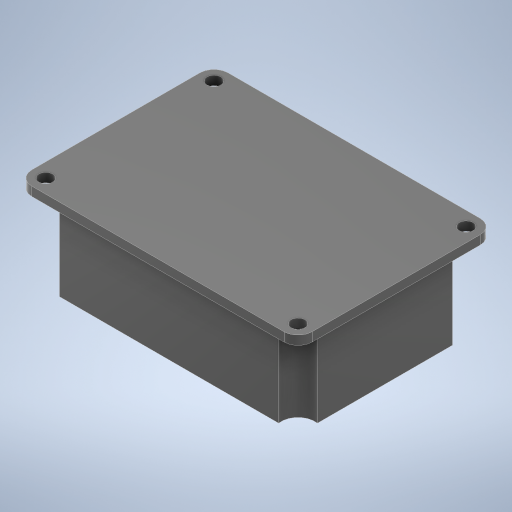
# Autodesk Inventor part: SUSTAINA-USB-AUDIO-BOARD
Saved by Autodesk Inventor 2024.2 (Build 282272000, 272)
## iProperties
Created: 2024-02-11
Part Number: SUSTAINA-USB-AUDIO-BOARD
Material: CFRP
Document SubType Name: Modeling
Designer: Masato Kubotera
Density: 1.43 g/cm^3
Appearance: Smooth - Black
Mass: 33.6504 g
Surface Area: 60.0346 cm^2
Volume: 23.5317 cm^3
Author: Masato Kubotera
Autodesk Inventor part; units mm, degrees
ref_plane "YZ Plane" through (0, 0, 0) normal (1, 0, 0) x (0, 1, 0)
ref_plane "XZ Plane" through (0, 0, 0) normal (0, 1, 0) x (-1, 0, 0)
ref_plane "XY Plane" through (0, 0, 0) normal (0, 0, 1) x (1, 0, 0)
sketch "Sketch1" plane through (0, 0, 0) normal (0, 0, 1) x (1, 0, 0)
  line L0 (17.5, 25) -> (-17.5, 25)
  line L1 (-17.5, 25) -> (-17.5, -25)
  line L2 (-17.5, -25) -> (17.5, -25)
  line L3 (17.5, -25) -> (17.5, 25)
  line L4 (17.5, 25) -> (-17.5, -25) construction
  line L5 (-17.5, 25) -> (17.5, -25) construction
  line L6 (-14, -18) -> (14, -18) construction
  line L7 (14, -18) -> (14, 18) construction
  line L8 (14, 18) -> (-14, 18) construction
  line L9 (-14, 18) -> (-14, -18) construction
  line L10 (-14, -18) -> (14, 18) construction
  line L11 (14, -18) -> (-14, 18) construction
  circle A0 centre (14, 18) radius 2.4 construction
  arc A1 (13.2801, 15.7105) -> (14.7199, 15.7105) centre (14, 15.5) ccw construction
  arc A2 (14.7199, 20.2895) -> (13.2801, 20.2895) centre (14, 20.5) ccw construction
  line L12 (0, 25) -> (0, -25) construction
  line L13 (17.5, 0) -> (-17.5, 0) construction
  line L14 (0, -25) -> (0, 25) construction
  line L15 (-15, -22.5) -> (15, -22.5) construction
  line L16 (15, -22.5) -> (15, 22.5) construction
  line L17 (15, 22.5) -> (-15, 22.5) construction
  line L18 (-15, 22.5) -> (-15, -22.5) construction
  line L19 (-15, -22.5) -> (15, 22.5) construction
  line L20 (15, -22.5) -> (-15, 22.5) construction
  circle A3 centre (15, 22.5) radius 2.5 construction
  arc A4 (12.042, 23) -> (15.5, 19.542) centre (15, 22.5) ccw
  line L21 (15.5, 19.542) -> (15.5, -19.542)
  line L22 (12.042, 23) -> (-12.042, 23)
  arc A5 (-15.5, 19.542) -> (-12.042, 23) centre (-15, 22.5) ccw
  line L23 (-15.5, 19.542) -> (-15.5, -19.542)
  arc A6 (15.5, -19.542) -> (12.042, -23) centre (15, -22.5) ccw
  line L24 (12.042, -23) -> (-12.042, -23)
  arc A7 (-12.042, -23) -> (-15.5, -19.542) centre (-15, -22.5) ccw
  point P0 (0, 0)
  point P1 (14, 14.75)
  point P2 (14, 21.25)
  point P3 (13.2801, 20.2895)
  point P4 (14.7199, 20.2895)
  dimension "d0" = 35
  dimension "d1" = 50
  dimension "d2" = 4.8
  dimension "d3" = 6.5
  dimension "d4" = 1.5
  dimension "d5" = 7
  dimension "d6" = 14
  dimension "d9" = 5
  dimension "d18" = 3
  dimension "d19" = 2
  dimension "d20" = 2
  constraints: 50 end point, 16 point on circle, 16 symmetric about line, 10 midpoint, 8 centre point, 7 coincident, 6 parallel, 4 horizontal, 3 perpendicular, 2 tangent, 1 point on line, 1 vertical, 4 other
  measures "d0" distance of L2.end L1.end
  measures "d1" distance of L1.end L0.end
  measures "d2" diameter of A0
  measures "d3" distance of point (14, 14.75) point (14, 21.25)
  measures "d4" diameter of A1
  measures "d5" diameter of L3 L7
  measures "d6" diameter of L0 L8
  measures "d9" diameter of A3
  measures "d18" radius of A4
  measures "d19" distance between parallel lines of L3 L21
  measures "d20" distance between parallel lines of L0 L22
extrude "Extrusion1" add sketch "Sketch1" along normal blind 1.6 contours L3 L2 L1 L0 | A4 L21 A6 L24 A7 L23 A5 L22
hole "Hole1" at (-15, -22.5, 0) at (-15, 22.5, 0) at (15, 22.5, 0) at (15, -22.5, 0) direction (0, 0, 1) diameter 2.5 end through all
fillet "Fillet1" radius 2.5 4 edges at (17.5, -25, 0.8) (-17.5, -25, 0.8) (-17.5, 25, 0.8) (17.5, 25, 0.8)
extrude "Extrusion2" add sketch "Sketch1" against normal blind 15 contours A4 L21 A6 L24 A7 L23 A5 L22
equation "\"d20\" = d19"
body "Solid1"
